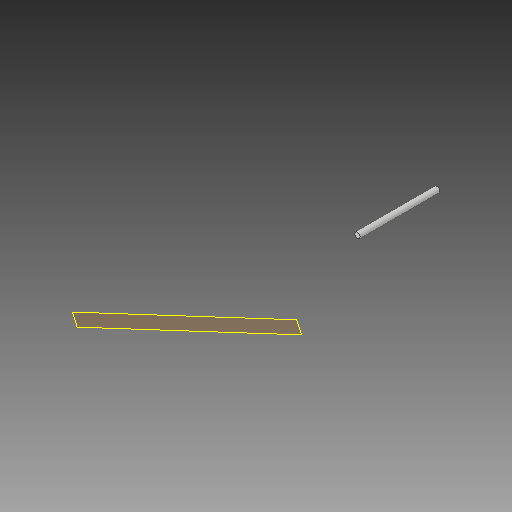
# Autodesk Inventor part: Part3
Saved by Autodesk Inventor 2017 (Build 210142000, 142)
## iProperties
Created: 2020-02-22
Part Number: Part3
Material: Generic
Document SubType Name: Modeling
Designer: S346553810
Density: 1 g/cm^3
Appearance: Default
Author: S346553810
Autodesk Inventor part; units mm, degrees
ref_plane "YZ Plane" through (0, 0, 0) normal (1, 0, 0) x (0, 1, 0)
ref_plane "XZ Plane" through (0, 0, 0) normal (0, 1, 0) x (-1, 0, 0)
ref_plane "XY Plane" through (0, 0, 0) normal (0, 0, 1) x (1, 0, 0)
ref_plane "Work Plane1" through (276.4709, -170.3537, 0) normal (0, 0, 1) x (-0.4255587, 0.9049308, 0)
sketch "Sketch1" plane through (276.4709, -170.3537, 0) normal (0, 0, 1) x (-0.4255587, 0.9049308, 0)
  circle A0 centre (189.1031, -168.3832) radius 6.35
  circle A1 centre (189.1031, -168.3832) radius 6.35
  point P0 (271.813, 177.6916)
  constraints: 2 centre point, 1 coincident, 1 concentric
ref_plane "Work Plane2" through (-239.4312, 84.6776, -190.5) normal (0, 0, 1) x (1, 0, 0)
extrude "Extrusion1" add sketch "Sketch1" against normal up to surface (190.5 mm away)
body "Solid1"
